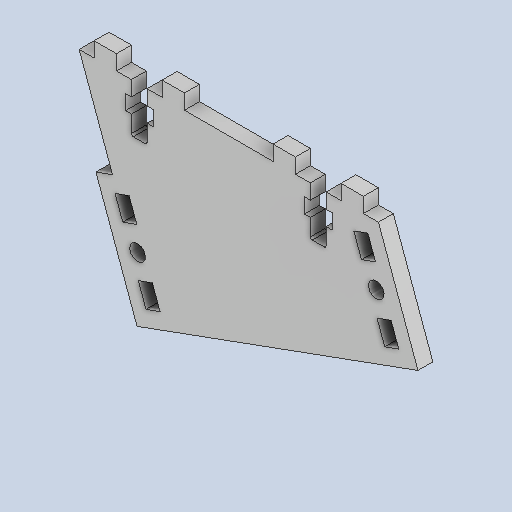
# Autodesk Inventor part: tc_support_front
Saved by Autodesk Inventor 2024.1 (Build 281209000, 209)
## iProperties
Created: 2019-07-16
Part Number: tc_support_front
Material: Acier inoxydable
Document SubType Name: Modeling
Designer: Thibault
Density: 8 g/cm^3
Appearance: Semi-poli
anchor_dist_b: 36.000 mm
anchor_dist_a: 2,000 mm
anchor_dist_top_a: 8.000 mm
tilt_angle: 20,00 deg
tc_plates_dist: 34,000 mm
Author: Thibault
Autodesk Inventor part; units mm, degrees
ref_plane "YZ Plane" through (0, 0, 0) normal (1, 0, 0) x (0, 1, 0)
ref_plane "XZ Plane" through (0, 0, 0) normal (0, 1, 0) x (-1, 0, 0)
ref_plane "XY Plane" through (0, 0, 0) normal (0, 0, 1) x (1, 0, 0)
sketch "Anchor (nut side)" plane through (0, 0, 0) normal (0, 0, 1) x (1, 0, 0)
  line L0 (11.1, 0) -> (9.1, 0)
  line L1 (9.1, 0) -> (9.1, -2)
  line L2 (9.1, -2) -> (9.9, -2)
  line L3 (9.9, -2) -> (9.9, -4)
  line L4 (6.2, -4) -> (6.2, -2)
  line L5 (6.2, -2) -> (7, -2)
  line L6 (7, -2) -> (7, 0)
  line L7 (7, 0) -> (5, 0)
  line L8 (2, 0) -> (2, 2)
  line L9 (2, 0) -> (3, 0) construction
  line L10 (2, 2) -> (5, 2)
  line L11 (5, 2) -> (5, 0)
  line L12 (11.1, 0) -> (11.1, 2)
  line L13 (11.1, 2) -> (14.1, 2)
  line L14 (14.1, 2) -> (14.1, 0)
  line L15 (0, 0) -> (2, 0)
  line L16 (14.1, 0) -> (16.1, 0)
  line L17 (6.2, -4) -> (7, -4)
  line L18 (9.9, -4) -> (9.1, -4)
  line L19 (7, -4) -> (7, -6.25)
  line L20 (9.1, -4) -> (9.1, -6.25)
  line L21 (7.25, -6.5) -> (8.05, -6.5)
  arc A0 (7, -6.25) -> (7.25, -6.5) centre (7.25, -6.25) ccw
  arc A1 (8.85, -6.5) -> (9.1, -6.25) centre (8.85, -6.25) ccw
  line L22 (8.05, -6.5) -> (8.85, -6.5)
  line L23 (8.05, -3.8983) -> (8.05, -9.959) construction
  point P0 (9.1321, -0.6227)
  point P1 (7, -6.5)
  point P2 (9.1, -6.5)
  dimension "d3" = 2
  dimension "d7" = 6.1
  dimension "d10" = 2
  dimension "d11" = 2
  dimension "d12" = 0.8
  dimension "d13" = 2
  dimension "d14" = 0.8
  dimension "d15" = 2.1
  dimension "d18" = 2
  dimension "d19" = 0.8
  dimension "d20" = 0.8
  dimension "d21" = 2.5
  dimension "d22" = 2.5
  dimension "d23" = 2.1
  dimension "d38" = 2
  dimension "d39" = 0.25
  dimension "d120" = 3
  measures "d3" distance of L15.start L8.start
  measures "d7" distance of L7.end L0.start
  measures "d10" distance of L0.start L0.end
  measures "d11" distance of L0.end L1.end
  measures "d12" distance of L1.end L2.end
  measures "d13" distance of L2.end L3.end
  measures "d14" distance of L4.end L5.end
  measures "d15" distance of L6.end L0.end
  measures "d18" distance of L14.end L16.end
  measures "d19" distance of L4.start L17.end
  measures "d20" distance of L3.end L18.end
  measures "d21" distance of L17.end point (7, -6.5)
  measures "d22" distance of L18.end point (9.1, -6.5)
  measures "d23" distance of L17.end L18.end
  measures "d38" distance between parallel lines of L15 L10
  measures "d39" radius of A0
  measures "d120" distance of L8.end L10.end
sketch "Anchor (screw side)" plane through (0, 0, 0) normal (0, 0, 1) x (1, 0, 0)
  circle A0 centre (93.8994, 50.2542) radius 1.05
  line L0 (90.8494, 51.2542) -> (87.8494, 51.2542)
  line L1 (87.8494, 51.2542) -> (87.8494, 49.2542)
  line L2 (87.8494, 49.2542) -> (90.8494, 49.2542)
  line L3 (90.8494, 49.2542) -> (90.8494, 51.2542)
  line L4 (99.9494, 51.2542) -> (96.9494, 51.2542)
  line L5 (96.9494, 51.2542) -> (96.9494, 49.2542)
  line L6 (96.9494, 49.2542) -> (99.9494, 49.2542)
  line L7 (99.9494, 49.2542) -> (99.9494, 51.2542)
  line L8 (90.8494, 51.2542) -> (96.9494, 49.2542) construction
  line L9 (96.9494, 51.2542) -> (90.8494, 49.2542) construction
  line L10 (85.8494, 53.2542) -> (101.9494, 53.2542) construction
  line L11 (101.9494, 53.2542) -> (101.9494, 47.2542) construction
  line L12 (101.9494, 47.2542) -> (85.8494, 47.2542) construction
  line L13 (85.8494, 47.2542) -> (85.8494, 53.2542) construction
  point P0 (103.5798, 50.1132)
  dimension "d27" = 2.1
  dimension "d28" = 3
  dimension "d29" = 2
  dimension "slot_distance" = 6.1
  dimension "d34" = 2
  dimension "d35_1" = 2
  dimension "d36_1" = 2
  dimension "d37" = 2
  measures "d27" diameter of A0
  measures "d28" distance of L2.end L1.end
  measures "d29" distance of L1.end L0.end
  measures "slot_distance" distance between parallel lines of L5 L3
  measures "d34" distance between parallel lines of L0 L10
  measures "d35_1" distance between parallel lines of L12 L2
  measures "d36_1" distance between parallel lines of L11 L7
  measures "d37" distance between parallel lines of L13 L1
derived "shared_parameters.ipt"
sketch "Esquisse1" plane through (0, 0, 0) normal (0, 0, 1) x (1, 0, 0)
  line L0 (82.7196, -31.2862) -> (77.4281, -16.7477)
  line L1 (82.7196, -31.2862) -> (47.3546, -44.158)
  line L2 (-2.0657, -1.8526) -> (7.9343, -1.7975) construction
  line L3 (41.8481, -29.029) -> (37.3781, -16.7477)
  line L4 (53.4781, -16.7477) -> (61.3281, -16.7477)
  line L5 (39.6254, -29.8379) -> (45.1319, -44.967)
  line L6 (39.6254, -29.8379) -> (41.8481, -29.029)
  line L7 (47.3546, -44.158) -> (47.3546, -44.158)
  line L8 (45.1319, -44.967) -> (47.3546, -44.158)
  circle A0 centre (77.1473, -24.7477) radius 1.05
  line L9 (77.2508, -27.9558) -> (78.2768, -30.7749)
  line L10 (78.2768, -30.7749) -> (80.1562, -30.0908)
  line L11 (80.1562, -30.0908) -> (79.1301, -27.2718)
  line L12 (79.1301, -27.2718) -> (77.2508, -27.9558)
  line L13 (74.1384, -19.4046) -> (75.1644, -22.2237)
  line L14 (75.1644, -22.2237) -> (77.0438, -21.5396)
  line L15 (77.0438, -21.5396) -> (76.0178, -18.7206)
  line L16 (76.0178, -18.7206) -> (74.1384, -19.4046)
  line L17 (77.2508, -27.9558) -> (77.0438, -21.5396) construction
  line L18 (75.1644, -22.2237) -> (79.1301, -27.2718) construction
  line L19 (77.0815, -33.3383) -> (71.5749, -18.2093) construction
  line L20 (71.5749, -18.2093) -> (77.2131, -16.1571) construction
  line L21 (77.2131, -16.1571) -> (82.7196, -31.2862) construction
  line L22 (82.7196, -31.2862) -> (77.0815, -33.3383) construction
  circle A1 centre (45.1977, -36.3764) radius 1.05
  line L23 (45.0943, -33.1683) -> (44.0682, -30.3492)
  line L24 (44.0682, -30.3492) -> (42.1888, -31.0333)
  line L25 (42.1888, -31.0333) -> (43.2149, -33.8524)
  line L26 (43.2149, -33.8524) -> (45.0943, -33.1683)
  line L27 (48.2067, -41.7195) -> (47.1806, -38.9004)
  line L28 (47.1806, -38.9004) -> (45.3012, -39.5845)
  line L29 (45.3012, -39.5845) -> (46.3273, -42.4036)
  line L30 (46.3273, -42.4036) -> (48.2067, -41.7195)
  line L31 (45.0943, -33.1683) -> (45.3012, -39.5845) construction
  line L32 (47.1806, -38.9004) -> (43.2149, -33.8524) construction
  line L33 (45.2636, -27.7858) -> (50.7701, -42.9149) construction
  line L34 (50.7701, -42.9149) -> (45.1319, -44.967) construction
  line L35 (45.1319, -44.967) -> (39.6254, -29.8379) construction
  line L36 (39.6254, -29.8379) -> (45.2636, -27.7858) construction
  line L37 (48.4781, -16.7477) -> (46.4781, -16.7477)
  line L38 (46.4781, -16.7477) -> (46.4781, -18.7477)
  line L39 (46.4781, -18.7477) -> (47.2781, -18.7477)
  line L40 (47.2781, -18.7477) -> (47.2781, -20.7477)
  line L41 (43.5781, -20.7477) -> (43.5781, -18.7477)
  line L42 (43.5781, -18.7477) -> (44.3781, -18.7477)
  line L43 (44.3781, -18.7477) -> (44.3781, -16.7477)
  line L44 (44.3781, -16.7477) -> (42.3781, -16.7477)
  line L45 (39.3781, -16.7477) -> (39.3781, -14.7477)
  line L46 (39.3781, -16.7477) -> (40.3781, -16.7477) construction
  line L47 (39.3781, -14.7477) -> (42.3781, -14.7477)
  line L48 (42.3781, -14.7477) -> (42.3781, -16.7477)
  line L49 (48.4781, -16.7477) -> (48.4781, -14.7477)
  line L50 (48.4781, -14.7477) -> (51.4781, -14.7477)
  line L51 (51.4781, -14.7477) -> (51.4781, -16.7477)
  line L52 (37.3781, -16.7477) -> (39.3781, -16.7477)
  line L53 (51.4781, -16.7477) -> (53.4781, -16.7477)
  line L54 (43.5781, -20.7477) -> (44.3781, -20.7477)
  line L55 (47.2781, -20.7477) -> (46.4781, -20.7477)
  line L56 (44.3781, -20.7477) -> (44.3781, -22.9977)
  line L57 (46.4781, -20.7477) -> (46.4781, -22.9977)
  line L58 (44.6281, -23.2477) -> (45.4281, -23.2477)
  arc A2 (44.3781, -22.9977) -> (44.6281, -23.2477) centre (44.6281, -22.9977) ccw
  arc A3 (46.2281, -23.2477) -> (46.4781, -22.9977) centre (46.2281, -22.9977) ccw
  line L59 (45.4281, -23.2477) -> (46.2281, -23.2477)
  line L60 (45.4281, -20.646) -> (45.4281, -26.7067) construction
  line L61 (72.4281, -16.7477) -> (70.4281, -16.7477)
  line L62 (70.4281, -16.7477) -> (70.4281, -18.7477)
  line L63 (70.4281, -18.7477) -> (71.2281, -18.7477)
  line L64 (71.2281, -18.7477) -> (71.2281, -20.7477)
  line L65 (67.5281, -20.7477) -> (67.5281, -18.7477)
  line L66 (67.5281, -18.7477) -> (68.3281, -18.7477)
  line L67 (68.3281, -18.7477) -> (68.3281, -16.7477)
  line L68 (68.3281, -16.7477) -> (66.3281, -16.7477)
  line L69 (63.3281, -16.7477) -> (63.3281, -14.7477)
  line L70 (63.3281, -16.7477) -> (64.3281, -16.7477) construction
  line L71 (63.3281, -14.7477) -> (66.3281, -14.7477)
  line L72 (66.3281, -14.7477) -> (66.3281, -16.7477)
  line L73 (72.4281, -16.7477) -> (72.4281, -14.7477)
  line L74 (72.4281, -14.7477) -> (75.4281, -14.7477)
  line L75 (75.4281, -14.7477) -> (75.4281, -16.7477)
  line L76 (61.3281, -16.7477) -> (63.3281, -16.7477)
  line L77 (75.4281, -16.7477) -> (77.4281, -16.7477)
  line L78 (67.5281, -20.7477) -> (68.3281, -20.7477)
  line L79 (71.2281, -20.7477) -> (70.4281, -20.7477)
  line L80 (68.3281, -20.7477) -> (68.3281, -22.9977)
  line L81 (70.4281, -20.7477) -> (70.4281, -22.9977)
  line L82 (68.5781, -23.2477) -> (69.3781, -23.2477)
  arc A4 (68.3281, -22.9977) -> (68.5781, -23.2477) centre (68.5781, -22.9977) ccw
  arc A5 (70.1781, -23.2477) -> (70.4281, -22.9977) centre (70.1781, -22.9977) ccw
  line L83 (69.3781, -23.2477) -> (70.1781, -23.2477)
  line L84 (69.3781, -20.646) -> (69.3781, -26.7067) construction
  point P0 (77.1473, -24.7477)
  point P1 (45.1977, -36.3764)
  dimension "d44" = 2
  dimension "d45" = 0.3653
  dimension "d55" = 40.05
  dimension "tc_plates_dist" = 34
  constraints: 18 end point, 3 horizontal, 2 perpendicular, 2 point on line, 1 collinear, 1 parallel, 14 other
  measures "d55" distance of L3.end L0.end
  measures "tc_plates_dist" distance of point (45.198, -36.376) point (77.147, -24.748)
extrude "Extrusion1" add sketch "Esquisse1" along normal blind 2
equation "\"d55\" = tc_base_back_width"
equation "\"d35\" = sheet_thickness"
equation "\"tc_base_back_width\" = 40.05"
equation "\"sheet_thickness\" = 2"
